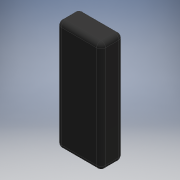
# Autodesk Inventor part: 升降板
Saved by Autodesk Inventor 2017 (Build 210142000, 142)
## iProperties
Part Number: 升降板
Material: 常规
Document SubType Name: Modeling
Designer: PANDA
Density: 1 g/cm^3
Appearance: 默认
Author: PANDA
Autodesk Inventor part; units mm, degrees
ref_plane "YZ Plane" through (0, 0, 0) normal (1, 0, 0) x (0, 1, 0)
ref_plane "XZ Plane" through (0, 0, 0) normal (0, 1, 0) x (-1, 0, 0)
ref_plane "XY Plane" through (0, 0, 0) normal (0, 0, 1) x (1, 0, 0)
sketch "草图1" plane through (0, 0, 0) normal (0, 1, 0) x (-1, 0, 0)
  line L0 (10, 25) -> (-10, 25)
  line L1 (-10, 25) -> (-10, -25)
  line L2 (-10, -25) -> (10, -25)
  line L3 (10, -25) -> (10, 25)
  point P0 (0, 0)
  dimension "d0" = 20
  dimension "d1" = 50
  constraints: 8 end point, 2 parallel, 1 horizontal, 1 perpendicular
  measures "d0" distance of L2.end L1.end
  measures "d1" distance of L1.end L0.end
extrude "拉伸1" add sketch "草图1" along normal blind 10
fillet "圆角1" radius 2 12 edges at (-10, 5, -25) (-10, 5, 25) (-10, 0, 0) (-10, 10, 0) (10, 5, -25) (0, 0, -25) (0, 10, -25) (10, 5, 25) (10, 0, 0) (10, 10, 0) (0, 0, 25) (0, 10, 25)
